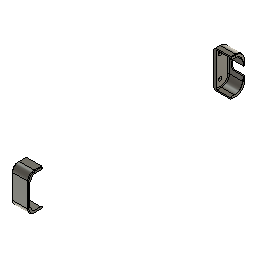
SKADIS_ExtentionCordMount (Autodesk Fusion 360 design; units mm, degrees)
Autodesk Fusion 360 part; units mm, degrees
sketch "SlotLayout" plane through (0, 0, 0) normal (1, 0, 0) x (0, 1, 0)
  line L0 (-22.4, 25) -> (-22.4, 15)
  line L1 (82.4, 5) -> (82.4, -5)
  line L2 (-37.6, -5) -> (-37.6, 5)
  line L3 (-80, 5) -> (-80, -5) construction
  line L4 (-97.6, 15) -> (-97.6, 25)
  line L5 (2.4, -5) -> (2.4, 5)
  arc A0 (-77.6, 5) -> (-82.4, 5) centre (-80, 5) ccw
  arc A1 (22.4, 25) -> (17.6, 25) centre (20, 25) ccw
  arc A2 (-97.6, 25) -> (-102.4, 25) centre (-100, 25) ccw
  arc A3 (97.6, 15) -> (102.4, 15) centre (100, 15) ccw
  line L6 (-60, 25) -> (-60, 15) construction
  line L7 (-77.6, -5) -> (-77.6, 5)
  arc A4 (77.6, -5) -> (82.4, -5) centre (80, -5) ccw
  line L8 (-40, 5) -> (-40, -5) construction
  line L9 (-57.6, 15) -> (-57.6, 25)
  line L10 (-62.4, 25) -> (-62.4, 15)
  line L11 (-102.4, 25) -> (-102.4, 15)
  line L12 (97.6, 15) -> (97.6, 25)
  arc A5 (-102.4, 15) -> (-97.6, 15) centre (-100, 15) ccw
  line L13 (20, 25) -> (20, 15) construction
  line L14 (22.4, 25) -> (22.4, 15)
  line L15 (-80, 0) -> (0, 0) construction
  line L16 (62.4, 25) -> (62.4, 15)
  line L17 (42.4, 5) -> (42.4, -5)
  arc A6 (2.5, 5) -> (-2.5, 5) centre (0, 5) ccw
  arc A7 (2.4, 5) -> (-2.4, 5) centre (0, 5) ccw
  line L18 (80, 5) -> (80, -5) construction
  arc A8 (82.4, 5) -> (77.6, 5) centre (80, 5) ccw
  arc A9 (-2.5, -5) -> (2.5, -5) centre (0, -5) ccw
  arc A10 (57.6, 15) -> (62.4, 15) centre (60, 15) ccw
  arc A11 (62.4, 25) -> (57.6, 25) centre (60, 25) ccw
  line L19 (17.6, 15) -> (17.6, 25)
  line L20 (-20, 25) -> (-20, 15) construction
  line L21 (-42.4, 5) -> (-42.4, -5)
  line L22 (60, 25) -> (60, 15) construction
  arc A12 (42.4, 5) -> (37.6, 5) centre (40, 5) ccw
  line L23 (-100, 25) -> (-100, 15) construction
  line L24 (100, 25) -> (100, 15) construction
  arc A13 (-57.6, 25) -> (-62.4, 25) centre (-60, 25) ccw
  arc A14 (37.6, -5) -> (42.4, -5) centre (40, -5) ccw
  line L25 (40, 5) -> (40, -5) construction
  line L26 (-17.6, 15) -> (-17.6, 25)
  arc A15 (-17.6, 25) -> (-22.4, 25) centre (-20, 25) ccw
  line L27 (-82.4, 5) -> (-82.4, -5)
  line L28 (-2.5, 5) -> (-2.5, -5)
  line L29 (-2.4, 5) -> (-2.4, -5)
  line L30 (102.4, 25) -> (102.4, 15)
  arc A16 (17.6, 15) -> (22.4, 15) centre (20, 15) ccw
  arc A17 (-22.4, 15) -> (-17.6, 15) centre (-20, 15) ccw
  line L31 (37.6, -5) -> (37.6, 5)
  line L32 (0, 5) -> (0, -5) construction
  arc A18 (-62.4, 15) -> (-57.6, 15) centre (-60, 15) ccw
  arc A19 (-42.4, -5) -> (-37.6, -5) centre (-40, -5) ccw
  arc A20 (-2.4, -5) -> (2.4, -5) centre (0, -5) ccw
  arc A21 (102.4, 25) -> (97.6, 25) centre (100, 25) ccw
  arc A22 (-82.4, -5) -> (-77.6, -5) centre (-80, -5) ccw
  arc A23 (-37.6, 5) -> (-42.4, 5) centre (-40, 5) ccw
  line L33 (77.6, -5) -> (77.6, 5)
  line L34 (57.6, 15) -> (57.6, 25)
  line L35 (2.5, -5) -> (2.5, 5)
  point P0 (-20, 20)
  point P1 (-40, 0)
  dimension "d9" = -40
  dimension "d10" = 0
  dimension "d255" = 0.1
  dimension "d22" = 10
  dimension "d23" = 2.4
  dimension "d4" = 40
  dimension "d25" = 40
  dimension "d26" = 20
  dimension "d27" = 20
  constraint tangent L27 A22
  constraint tangent L7 A22
  constraint parallel L7 L27
  constraint tangent A0 L7
  constraint tangent A0 L27
  constraint vertical L3
  constraint tangent L21 A19
  constraint tangent L2 A19
  constraint parallel L2 L21
  constraint tangent L2 A23
  constraint tangent L21 A23
  constraint vertical L8
  constraint tangent L29 A20
  constraint tangent L5 A20
  constraint parallel L5 L29
  constraint tangent L5 A7
  constraint tangent A7 L29
  constraint parallel L2 L32
  constraint midpoint L15.start L3
  constraint midpoint L15.end L32
  constraint horizontal L15
  constraint equal L8 L32
  constraint equal L3 L8
  constraint midpoint P1 L8
  constraint coincident P1 L15
  constraint equal A7 A23
  constraint equal A0 A23
  constraint coincident L15.end origin
  constraint symmetric A0.end L1.start L32
  constraint symmetric L1.end L27.end L32
  constraint symmetric L7.start A4.start L32
  constraint symmetric A8.end A0.start L32
  constraint symmetric A4 L32 A22
  constraint symmetric A0 A8 L32
  constraint symmetric L17.start L21.start L32
  constraint symmetric L17.end L21.end L32
  constraint symmetric A14.start L2.start L32
  constraint symmetric A12.end L2.end L32
  constraint symmetric A14 L32 A19
  constraint symmetric A12 L32 A23
  constraint tangent L0 A17
  constraint tangent L26 A17
  constraint parallel L0 L26
  constraint tangent L26 A15
  constraint tangent L0 A15
  constraint vertical L20
  constraint equal L20 L32
  constraint equal A7 A15
  constraint midpoint P0 L20
  constraint symmetric L0.end L14.end L32
  constraint symmetric L26.end A1.end L32
  constraint symmetric L0.start A1.start L32
  constraint symmetric L26.start L19.start L32
  constraint symmetric A1 A15 L32
  constraint symmetric A16 A17 L32
  constraint symmetric A11.end L9.end L32
  constraint symmetric L16.start L10.start L32
  constraint symmetric A11 A13 L32
  constraint symmetric L16.end L10.end L32
  constraint symmetric A10.start L9.start L32
  constraint symmetric A10 L32 A18
  constraint symmetric L12.end L4.end L32
  constraint symmetric L30.start A2.end L32
  constraint symmetric A2 L32 A21
  constraint symmetric A3.end L11.end L32
  constraint symmetric A3.start L4.start L32
  constraint symmetric A3 A5 L32
  measures "d22" distance of A6.centre A9.centre
  measures "d23" radius of A7
  measures "d4" distance of L8 L32
  measures "d25" distance of L3 L8
  measures "d26" horizontal distance of L20.end A6.centre
  measures "d27" vertical distance of P0 L15.end
sketch "PrintKey" plane through (0, 0, 0) normal (1, 0, 0) x (0, 1, 0)
  circle A0 centre (0, 0) radius 1.6
  line L0 (2.6, -6.7) -> (-2.6, -6.7)
  line L1 (-2.6, -6.7) -> (-2.6, 6.7)
  line L2 (-2.6, 6.7) -> (2.6, 6.7)
  line L3 (2.6, 6.7) -> (2.6, -6.7)
  line L4 (0, 6.7) -> (0, -6.7) construction
  line L5 (0, 6.7) -> (0, 23.5939) construction
  line L6 (0, 23.5939) -> (-8.4469, 15.1469) construction
  line L7 (-8.4469, 15.1469) -> (8.4469, 15.1469) construction
  line L8 (8.4469, 15.1469) -> (0, 23.5939) construction
  circle A1 centre (0, 0) radius 3.4
  line L9 (17.4, -6.7) -> (17.4, 6.7)
  line L10 (22.6, -6.7) -> (17.4, -6.7)
  line L11 (22.6, 6.7) -> (22.6, -6.7)
  line L12 (17.4, 6.7) -> (22.6, 6.7)
  circle A2 centre (20, 0) radius 1.6
  circle A3 centre (20, 0) radius 3.4
  line L13 (20, 6.7) -> (20, -6.7) construction
  line L14 (37.4, -6.7) -> (37.4, 6.7)
  line L15 (42.6, -6.7) -> (37.4, -6.7)
  line L16 (42.6, 6.7) -> (42.6, -6.7)
  line L17 (37.4, 6.7) -> (42.6, 6.7)
  circle A4 centre (40, 0) radius 1.6
  circle A5 centre (40, 0) radius 3.4
  line L18 (40, 6.7) -> (40, -6.7) construction
  line L19 (57.4, -6.7) -> (57.4, 6.7)
  line L20 (62.6, -6.7) -> (57.4, -6.7)
  line L21 (62.6, 6.7) -> (62.6, -6.7)
  line L22 (57.4, 6.7) -> (62.6, 6.7)
  circle A6 centre (60, 0) radius 1.6
  circle A7 centre (60, 0) radius 3.4
  line L23 (60, 6.7) -> (60, -6.7) construction
  line L24 (-22.6, -6.7) -> (-22.6, 6.7)
  line L25 (-22.6, 6.7) -> (-17.4, 6.7)
  line L26 (-17.4, -6.7) -> (-22.6, -6.7)
  line L27 (-17.4, 6.7) -> (-17.4, -6.7)
  line L28 (-20, 6.7) -> (-20, -6.7) construction
  circle A8 centre (-20, 0) radius 3.4
  circle A9 centre (-20, 0) radius 1.6
  line L29 (-42.6, -6.7) -> (-42.6, 6.7)
  line L30 (-42.6, 6.7) -> (-37.4, 6.7)
  line L31 (-37.4, -6.7) -> (-42.6, -6.7)
  line L32 (-37.4, 6.7) -> (-37.4, -6.7)
  line L33 (-40, 6.7) -> (-40, -6.7) construction
  circle A10 centre (-40, 0) radius 3.4
  circle A11 centre (-40, 0) radius 1.6
  line L34 (-62.6, -6.7) -> (-62.6, 6.7)
  line L35 (-62.6, 6.7) -> (-57.4, 6.7)
  line L36 (-57.4, -6.7) -> (-62.6, -6.7)
  line L37 (-57.4, 6.7) -> (-57.4, -6.7)
  line L38 (-60, 6.7) -> (-60, -6.7) construction
  circle A12 centre (-60, 0) radius 3.4
  circle A13 centre (-60, 0) radius 1.6
  line L39 (-82.6, -6.7) -> (-82.6, 6.7)
  line L40 (-82.6, 6.7) -> (-77.4, 6.7)
  line L41 (-77.4, -6.7) -> (-82.6, -6.7)
  line L42 (-77.4, 6.7) -> (-77.4, -6.7)
  line L43 (-80, 6.7) -> (-80, -6.7) construction
  circle A14 centre (-80, 0) radius 3.4
  circle A15 centre (-80, 0) radius 1.6
  line L44 (-102.6, -6.7) -> (-102.6, 6.7)
  line L45 (-102.6, 6.7) -> (-97.4, 6.7)
  line L46 (-97.4, -6.7) -> (-102.6, -6.7)
  line L47 (-97.4, 6.7) -> (-97.4, -6.7)
  line L48 (-100, 6.7) -> (-100, -6.7) construction
  circle A16 centre (-100, 0) radius 3.4
  circle A17 centre (-100, 0) radius 1.6
  line L49 (-122.6, -6.7) -> (-122.6, 6.7)
  line L50 (-122.6, 6.7) -> (-117.4, 6.7)
  line L51 (-117.4, -6.7) -> (-122.6, -6.7)
  line L52 (-117.4, 6.7) -> (-117.4, -6.7)
  line L53 (-120, 6.7) -> (-120, -6.7) construction
  circle A18 centre (-120, 0) radius 3.4
  circle A19 centre (-120, 0) radius 1.6
  line L54 (-142.6, -6.7) -> (-142.6, 6.7)
  line L55 (-142.6, 6.7) -> (-137.4, 6.7)
  line L56 (-137.4, -6.7) -> (-142.6, -6.7)
  line L57 (-137.4, 6.7) -> (-137.4, -6.7)
  line L58 (-140, 6.7) -> (-140, -6.7) construction
  circle A20 centre (-140, 0) radius 3.4
  circle A21 centre (-140, 0) radius 1.6
  line L59 (-162.6, -6.7) -> (-162.6, 6.7)
  line L60 (-162.6, 6.7) -> (-157.4, 6.7)
  line L61 (-157.4, -6.7) -> (-162.6, -6.7)
  line L62 (-157.4, 6.7) -> (-157.4, -6.7)
  line L63 (-160, 6.7) -> (-160, -6.7) construction
  circle A22 centre (-160, 0) radius 3.4
  circle A23 centre (-160, 0) radius 1.6
  line L64 (-182.6, -6.7) -> (-182.6, 6.7)
  line L65 (-182.6, 6.7) -> (-177.4, 6.7)
  line L66 (-177.4, -6.7) -> (-182.6, -6.7)
  line L67 (-177.4, 6.7) -> (-177.4, -6.7)
  line L68 (-180, 6.7) -> (-180, -6.7) construction
  circle A24 centre (-180, 0) radius 3.4
  circle A25 centre (-180, 0) radius 1.6
  line L69 (77.4, -6.7) -> (77.4, 6.7)
  line L70 (82.6, -6.7) -> (77.4, -6.7)
  line L71 (82.6, 6.7) -> (82.6, -6.7)
  line L72 (77.4, 6.7) -> (82.6, 6.7)
  circle A26 centre (80, 0) radius 1.6
  circle A27 centre (80, 0) radius 3.4
  line L73 (80, 6.7) -> (80, -6.7) construction
  line L74 (97.4, -6.7) -> (97.4, 6.7)
  line L75 (102.6, -6.7) -> (97.4, -6.7)
  line L76 (102.6, 6.7) -> (102.6, -6.7)
  line L77 (97.4, 6.7) -> (102.6, 6.7)
  circle A28 centre (100, 0) radius 1.6
  circle A29 centre (100, 0) radius 3.4
  line L78 (100, 6.7) -> (100, -6.7) construction
  line L79 (117.4, -6.7) -> (117.4, 6.7)
  line L80 (122.6, -6.7) -> (117.4, -6.7)
  line L81 (122.6, 6.7) -> (122.6, -6.7)
  line L82 (117.4, 6.7) -> (122.6, 6.7)
  circle A30 centre (120, 0) radius 1.6
  circle A31 centre (120, 0) radius 3.4
  line L83 (120, 6.7) -> (120, -6.7) construction
  line L84 (137.4, -6.7) -> (137.4, 6.7)
  line L85 (142.6, -6.7) -> (137.4, -6.7)
  line L86 (142.6, 6.7) -> (142.6, -6.7)
  line L87 (137.4, 6.7) -> (142.6, 6.7)
  circle A32 centre (140, 0) radius 1.6
  circle A33 centre (140, 0) radius 3.4
  line L88 (140, 6.7) -> (140, -6.7) construction
  line L89 (157.4, -6.7) -> (157.4, 6.7)
  line L90 (162.6, -6.7) -> (157.4, -6.7)
  line L91 (162.6, 6.7) -> (162.6, -6.7)
  line L92 (157.4, 6.7) -> (162.6, 6.7)
  circle A34 centre (160, 0) radius 1.6
  circle A35 centre (160, 0) radius 3.4
  line L93 (160, 6.7) -> (160, -6.7) construction
  line L94 (177.4, -6.7) -> (177.4, 6.7)
  line L95 (182.6, -6.7) -> (177.4, -6.7)
  line L96 (182.6, 6.7) -> (182.6, -6.7)
  line L97 (177.4, 6.7) -> (182.6, 6.7)
  circle A36 centre (180, 0) radius 1.6
  circle A37 centre (180, 0) radius 3.4
  line L98 (180, 6.7) -> (180, -6.7) construction
  line L99 (-157.4, -13.3) -> (-157.4, -26.7)
  line L100 (-160, -13.3) -> (-160, -26.7) construction
  line L101 (-157.4, -26.7) -> (-162.6, -26.7)
  circle A38 centre (-160, -20) radius 1.6
  circle A39 centre (-160, -20) radius 3.4
  line L102 (-162.6, -13.3) -> (-157.4, -13.3)
  line L103 (-162.6, -26.7) -> (-162.6, -13.3)
  line L104 (160, -13.3) -> (160, -26.7) construction
  circle A40 centre (160, -20) radius 1.6
  line L105 (157.4, -26.7) -> (157.4, -13.3)
  line L106 (162.6, -26.7) -> (157.4, -26.7)
  line L107 (157.4, -13.3) -> (162.6, -13.3)
  circle A41 centre (160, -20) radius 3.4
  line L108 (162.6, -13.3) -> (162.6, -26.7)
  line L109 (177.4, -33.3) -> (182.6, -33.3)
  line L110 (182.6, -46.7) -> (177.4, -46.7)
  line L111 (182.6, -33.3) -> (182.6, -46.7)
  circle A42 centre (180, -40) radius 1.6
  circle A43 centre (180, -40) radius 3.4
  line L112 (180, -33.3) -> (180, -46.7) construction
  line L113 (177.4, -46.7) -> (177.4, -33.3)
  line L114 (-177.4, -46.7) -> (-182.6, -46.7)
  line L115 (-182.6, -33.3) -> (-177.4, -33.3)
  line L116 (-182.6, -46.7) -> (-182.6, -33.3)
  line L117 (-177.4, -33.3) -> (-177.4, -46.7)
  circle A44 centre (-180, -40) radius 1.6
  line L118 (-180, -33.3) -> (-180, -46.7) construction
  circle A45 centre (-180, -40) radius 3.4
  point P0 (20, 0)
  point P1 (20, 0)
  point P2 (20, 0)
  point P3 (40, 0)
  point P4 (40, 0)
  point P5 (40, 0)
  point P6 (60, 0)
  point P7 (60, 0)
  point P8 (60, 0)
  point P9 (80, 0)
  point P10 (80, 0)
  point P11 (80, 0)
  point P12 (100, 0)
  point P13 (100, 0)
  point P14 (100, 0)
  point P15 (120, 0)
  point P16 (120, 0)
  point P17 (120, 0)
  point P18 (140, 0)
  point P19 (140, 0)
  point P20 (140, 0)
  point P21 (160, 0)
  point P22 (160, 0)
  point P23 (160, 0)
  point P24 (180, 0)
  point P25 (180, 0)
  point P26 (180, 0)
  point P27 (160, -20)
  point P28 (160, -20)
  point P29 (160, -20)
  point P30 (180, -40)
  point P31 (180, -40)
  point P32 (180, -40)
  dimension "d21" = 13.4
  dimension "d24" = 5.2
  dimension "d28" = 3.2
  dimension "d34" = 6.8
  dimension "d37" = 20
  dimension "d38" = 0
  dimension "d41" = -20
  dimension "d42" = 0
  dimension "d84" = 0
  dimension "d85" = -20
  dimension "d88" = 0
  dimension "d89" = -40
  constraint horizontal L2
  constraint vertical L3
  constraint horizontal L0
  constraint vertical L1
  constraint midpoint L4.start L2
  constraint midpoint L4.end L0
  constraint midpoint A0.centre L4
  constraint coincident A0.centre A1.centre
  constraint perpendicular L2 L5
  constraint perpendicular L5 L7
  constraint midpoint L5 L7
  constraint perpendicular L6 L8
  measures "d21" distance of L4.end L4.start
  measures "d24" distance of L1 L3
  measures "d28" diameter of A0
  measures "d34" diameter of A1
sketch "Sketch1" plane through (0, 0, 0) normal (1, 0, 0) x (0, 1, 0) in component "ExtentsionSocketMount_Left"
  line L0 (-186, 9) -> (181, 9) construction
  line L1 (195, -5) -> (195, -39) construction
  line L2 (181, -53) -> (-186, -53) construction
  line L3 (-195, -44) -> (-195, 0) construction
  line L4 (-195, -22) -> (195, -22) construction
  arc A0 (-186, 9) -> (-195, 0) centre (-186, 0) ccw construction
  arc A1 (-195, -44) -> (-186, -53) centre (-186, -44) ccw construction
  arc A2 (195, -5) -> (181, 9) centre (181, -5) ccw construction
  arc A3 (181, -53) -> (195, -39) centre (181, -39) ccw construction
  arc A4 (-186, 9.4) -> (-195.4, 0) centre (-186, 0) ccw
  line L5 (-195.4, -44) -> (-195.4, 0)
  arc A5 (-195.4, -44) -> (-186, -53.4) centre (-186, -44) ccw
  line L6 (-186, -53.4) -> (-172.8, -53.4)
  line L7 (-186, 9.4) -> (-172.8, 9.4)
  arc A6 (-193, -44) -> (-186, -51) centre (-186, -44) ccw
  line L8 (-193, -44) -> (-195.4, -41.6)
  line L9 (-186, -51) -> (-172.8, -51)
  line L10 (-172.8, -55.8) -> (-186, -55.8)
  arc A7 (-197.8, -44) -> (-186, -55.8) centre (-186, -44) ccw
  line L11 (-132.8, 11.8) -> (-132.8, -9)
  line L12 (-172.8, 11.8) -> (-132.8, 11.8)
  arc A8 (-186, 11.8) -> (-197.8, 0) centre (-186, 0) ccw
  arc A9 (-186, 7) -> (-193, 0) centre (-186, 0) ccw
  line L13 (-193, 0) -> (-195.4, -2.4)
  line L14 (-186, 7) -> (-172.8, 7)
  line L15 (-172.8, 11.8) -> (-186, 11.8)
  line L16 (-197.8, 0) -> (-197.8, -44)
  line L17 (-172.8, -55.8) -> (-172.8, 11.8)
  line L18 (-172.8, 7) -> (-132.8, 7)
  line L19 (-172.8, 9.4) -> (-132.8, 9.4)
  line L20 (-132.8, -9) -> (-132.8, -55.8)
  line L21 (-172.8, -55.8) -> (-132.8, -55.8)
  line L22 (-172.8, -51) -> (-132.8, -51)
  line L23 (-172.8, -53.4) -> (-132.8, -53.4)
  line L24 (-132.8, -9) -> (-159.82, -55.8)
  line L25 (172.8, 12.4529) -> (172.8, -55.8)
  arc A10 (181, -53.4) -> (195.4, -39) centre (181, -39) ccw
  line L26 (195.4, -5) -> (195.4, -39)
  arc A11 (181, -55.8) -> (197.8, -39) centre (181, -39) ccw
  line L27 (197.8, -5) -> (197.8, -39)
  line L28 (181, -53.4) -> (172.8, -53.4)
  line L29 (181, -55.8) -> (172.8, -55.8)
  arc A12 (181, -51) -> (193, -39) centre (181, -39) ccw
  line L30 (193, -39) -> (195.4, -36.6)
  line L31 (181, -51) -> (172.8, -51)
  line L32 (195.4, -22) -> (197.8, -22) construction
  line L33 (197.8, -30) -> (195.4, -30)
  line L34 (197.8, -14) -> (195.4, -14)
  arc A13 (197.8, -5) -> (181, 11.8) centre (181, -5) ccw
  arc A14 (195.4, -5) -> (181, 9.4) centre (181, -5) ccw
  arc A15 (193, -5) -> (181, 7) centre (181, -5) ccw
  line L35 (193, -5) -> (195.4, -7.4)
  line L36 (181, 7) -> (172.8, 7)
  line L37 (181, 9.4) -> (172.8, 9.4)
  line L38 (181, 11.8) -> (172.8, 11.8)
  point P0 (0, -22)
  point P1 (-180, 0)
  point P2 (-160, 0)
  point P3 (-160, 0)
  point P4 (-140, 0)
  dimension "d43" = 390
  dimension "d44" = 62
  dimension "d45" = 22
  dimension "d46" = 9
  dimension "d47" = 14
  dimension "d48" = 0.4
  dimension "d50" = 45
  dimension "d51" = 2.4
  dimension "d52" = 2.4
  dimension "d61" = 25
  dimension "d62" = 9
  dimension "d75" = 40
  dimension "d76" = 30
  dimension "d96" = 2.4
  dimension "d98" = 2.4
  dimension "d99" = 25
  dimension "d100" = 8
  constraint horizontal L0
  constraint vertical L1
  constraint horizontal L2
  constraint vertical L3
  constraint perpendicular L1 L4
  constraint midpoint L4 P0
  constraint vertical origin P0
  constraint coincident L3 L4.start
  constraint tangent L0 A0
  constraint tangent L3 A0
  constraint tangent L3 A1
  constraint tangent L2 A1
  constraint equal A0 A1
  constraint coincident L1 L4.end
  constraint tangent L0 A2
  constraint tangent L1 A2
  constraint tangent L1 A3
  constraint tangent L2 A3
  constraint equal A2 A3
  constraint midpoint L1 L4.end
  constraint tangent A5 L6
  constraint parallel L2 L6
  constraint coincident L5 L8.end
  constraint concentric A1 A6
  constraint tangent A6 L9
  constraint horizontal A1.centre A6.start
  constraint tangent L10 A7
  constraint concentric A1 A7
  constraint perpendicular L4 L11
  constraint symmetric L4 A6.start A9.end
  constraint symmetric L4 A6.end A9.start
  constraint symmetric L4 A6 A9
  constraint symmetric L4 L8.end L13.end
  constraint symmetric L4 L9.end L14.end
  constraint symmetric L4 L10.start L12.start
  constraint symmetric L4 L10.end A8.start
  constraint symmetric L4 A7.start A8.end
  constraint symmetric L4 A7 A8
  constraint perpendicular L12 L17
  constraint coincident L7.end L17
  constraint perpendicular L7 L17
  constraint coincident L6.end L17
  constraint coincident L9.end L17
  constraint tangent A7 L16
  constraint coincident L11 L18.end
  constraint perpendicular L11 L18
  constraint coincident L11 L19.end
  constraint perpendicular L11 L19
  constraint perpendicular L2 L20
  constraint coincident L20 L22.end
  constraint perpendicular L20 L22
  constraint coincident L20 L23.end
  constraint perpendicular L20 L23
  constraint perpendicular L20 L21
  constraint coincident L21 L24.end
  constraint perpendicular L2 L25
  constraint coincident L25 L28.end
  constraint tangent A10 L28
  constraint perpendicular L25 L28
  constraint coincident L25 L29.end
  constraint tangent A11 L29
  constraint perpendicular L25 L29
  constraint coincident L25 L25.start
  constraint concentric A3 A12
  constraint coincident L26 L30.end
  constraint coincident L25 L31.end
  constraint tangent A12 L31
  constraint perpendicular L25 L31
  constraint perpendicular L8 L30
  constraint horizontal A3.centre A12.end
  constraint concentric A3 A11
  constraint concentric A3 A10
  constraint vertical L27
  constraint tangent A11 L27
  constraint midpoint L26 L32.start
  constraint midpoint L27 L32.end
  constraint horizontal L4.end L32.start
  constraint horizontal L32
  constraint coincident L27 L33.start
  constraint perpendicular L27 L33
  constraint coincident L26 L33.end
  constraint symmetric L4 A10.end L26.start
  constraint symmetric L4 A10.start A14.end
  constraint symmetric L4 A10 A14
  constraint symmetric L4 A11.end L27.start
  constraint symmetric L4 A11.start A13.end
  constraint symmetric L4 A11 A13
  constraint symmetric L4 L28.end L37.end
  constraint symmetric L4 L25.end L38.end
  constraint symmetric L4 A12.end A15.start
  constraint symmetric L4 A12.start A15.end
  constraint symmetric L4 A12 A15
  constraint symmetric L4 L30.end L35.end
  constraint symmetric L4 L31.end L36.end
  constraint symmetric L4 L33.start L34.start
  constraint symmetric L4 L33.end L34.end
  measures "d43" distance of L4.start L4.end
  measures "d44" distance of L0 L2
  measures "d45" distance of P0 origin
  measures "d46" radius of A0
  measures "d47" radius of A2
  measures "d50" angle of L5 L8
  measures "d51" distance of L6 L9
  measures "d52" distance of L6 L10
  measures "d61" distance of L16 L17
  measures "d62" vertical distance of L11.end P3
  measures "d75" distance of L11 L17
  measures "d76" angle of L20 L24
  measures "d96" distance of L28 L31
  measures "d98" distance of A10 A11
  measures "d99" distance of L25 L27
  measures "d100" distance of L32 L33
extrude "Extrude1" add sketch "Sketch1" along normal blind 4 contours A4 L5 L7 A9 L13 L14 L17 | A4 L5 A5 L6 L7 L10 A7 A8 L15 L16 L17 | L11 L17 L18 L19 | L11 L12 L17 L19 | L5 A6 L8 L9 A9 L13 L14 L17 | L11 L17 L18 L22 L24 | L5 A5 L6 A6 L8 L9 L17 | L17 L22 L23 L24 | L17 L21 L23 L24 | L25 L26 L27 L34 A13 A14 L37 L38 | L25 L26 A14 A15 L35 L36 L37 | L25 L26 A12 L30 L31 A15 L35 L36 | L25 A10 L26 L28 A12 L30 L31 | L26 L27 L33 L34 | L25 A10 L26 A11 L27 L28 L29 L33 makes body 1 at (0, -163.4733, -21.6) makes body 2 at (0, 181.1333, -16.3333) in component "ExtentsionSocketMount_Left"
extrude "Extrude2" add sketch "Sketch1" along normal blind 25.2 from surface at 4 contours A4 L5 A5 L6 L7 L10 A7 A8 L15 L16 L17 | L11 L12 L17 L19 | L17 L21 L23 L24 | L25 L26 L27 L34 A13 A14 L37 L38 | L25 A10 L26 A11 L27 L28 L29 L33 bodies 1 2 in component "ExtentsionSocketMount_Left"
extrude "Extrude3" add sketch "Sketch1" along normal blind 2.4 from surface at 29.2 contours A4 L5 L7 A9 L13 L14 L17 | A4 L5 A5 L6 L7 L10 A7 A8 L15 L16 L17 | L11 L17 L18 L19 | L11 L12 L17 L19 | L5 A5 L6 A6 L8 L9 L17 | L17 L22 L23 L24 | L17 L21 L23 L24 | L25 L26 L27 L34 A13 A14 L37 L38 | L25 L26 A14 A15 L35 L36 L37 | L25 A10 L26 L28 A12 L30 L31 | L25 A10 L26 A11 L27 L28 L29 L33 bodies 1 2 in component "ExtentsionSocketMount_Left"
extrude "Extrude7" add sketch "Sketch1" along normal blind 5 from surface at 4 contours L26 L27 L33 L34 bodies 2 in component "ExtentsionSocketMount_Left"
chamfer "Chamfer1" distance 2.4 angle 45 4 edges at (29.2, -159.4, 7) (29.2, -190.9497, 4.9497) (29.2, -171.5244, -51) (29.2, -190.9497, -48.9497) on bodies 1 in component "ExtentsionSocketMount_Left"
chamfer "Chamfer1" distance 1.5 angle 45 5 edges at (4, -159.4, 9.4) (4, -192.6468, 6.6468) (4, -195.4, -22) (4, -192.6468, -50.6468) (4, -172.2172, -53.4) on bodies 1 in component "ExtentsionSocketMount_Left"
chamfer "Chamfer5" distance 2.4 angle 45 4 edges at (29.2, 189.4853, -47.4853) (29.2, 176.9, -51) (29.2, 189.4853, 3.4853) (29.2, 176.9, 7) on bodies 2 in component "ExtentsionSocketMount_Left"
chamfer "Chamfer5" distance 1.5 angle 45 5 edges at (4, 195.4, -22) (4, 191.1823, -49.1823) (4, 176.9, -53.4) (4, 176.9, 9.4) (4, 191.1823, 5.1823) on bodies 2 in component "ExtentsionSocketMount_Left"
chamfer "Chamfer5" distance 3 angle 45 5 edges at (0, 176.9, 11.8) (0, 176.9, -55.8) (0, 192.8794, -50.8794) (0, 197.8, -22) (0, 192.8794, 6.8794) on bodies 2 in component "ExtentsionSocketMount_Left"
chamfer "Chamfer5" distance 1 angle 45 6 edges at (31.6, 192.8794, 6.8794) (31.6, 176.9, 11.8) (31.6, 197.8, -9.5) (31.6, 192.8794, -50.8794) (31.6, 197.8, -34.5) (31.6, 176.9, -55.8) on bodies 2 in component "ExtentsionSocketMount_Left"
chamfer "Chamfer2" distance 3 angle 45 5 edges at (0, -159.4, 11.8) (0, -194.3439, 8.3439) (0, -197.8, -22) (0, -194.3439, -52.3439) (0, -172.91, -55.8) on bodies 1 in component "ExtentsionSocketMount_Left"
fillet "Fillet1" radius 6 2 edges at (9, 196.6, -30) (9, 196.6, -14) on bodies 2 in component "ExtentsionSocketMount_Left"
extrude "Extrude4" cut sketch "PrintKey" along normal blind 1.8 contours L54 L56 L57 A20 | L54 L57 A20 | L54 L55 L57 A20 | A21 | L64 L66 L67 A24 | L64 L67 A24 | L64 L65 L67 A24 | A25 | L94 L95 L96 A37 | L94 L96 A37 | L94 L96 L97 A37 | A36 | L109 L111 A43 L113 | L111 A43 L113 | L110 L111 A43 L113 | A42 | L114 L116 L117 A45 | L116 L117 A45 | L115 L116 L117 A45 | A44 bodies 1 2 in component "ExtentsionSocketMount_Left"
extrude "Extrude5" cut sketch "PrintKey" along normal through all contours A21 | A25 | A36 | A42 | A44 bodies 1 2 in component "ExtentsionSocketMount_Left"
chamfer "Chamfer3" distance 1.8 angle 45 5 edges at (4, 178.5083, 0.5786) (4, 178.5083, -39.4214) (4, -141.4917, 0.5786) (4, -181.4917, 0.5786) (4, -181.4917, -39.4214) on bodies 1 2 in component "ExtentsionSocketMount_Left"
chamfer "Chamfer4" distance 1 angle 45 5 edges at (31.6, -172.91, -55.8) (31.6, -197.8, -22) (31.6, -194.3439, -52.3439) (31.6, -194.3439, 8.3439) (31.6, -159.4, 11.8) on bodies 1 in component "ExtentsionSocketMount_Left"
extrude "Extrude6" cut sketch "Sketch1" along normal blind 68 contours L11 L17 L18 L19 | L11 L12 L17 L19 | L11 L17 L18 L22 L24 | L17 L22 L23 L24 | L17 L21 L23 L24 bodies 1 in component "ExtentsionSocketMount_Left"
component "ExtentsionSocketMount_Left" placed x (1, 0, 0) y (0, 1, 0) z (0, 0, 1) at (0, 0, 0)
equation "XY_Tolerance = 0.2 mm"
equation "Z_Tolerance = 0.2 mm"
equation "Wall_Thickness = 0.4 mm"
equation "Layer_Height = 0.2 mm"
equation "M3Hole_wClearance = 3.2 mm"
equation "M3Hole_wSelfTapping = 2.8 mm"
equation "d28 = M3Hole_wClearance"
equation "M3Hole_CounterSink = 1.8 mm"
equation "d48 = XY_Tolerance * 2"
equation "d67 = 25 mm + XY_Tolerance"
equation "d80 = M3Hole_CounterSink"
